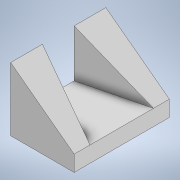
# Autodesk Inventor part: 零件9
Saved by Autodesk Inventor 2020 (Build 240168000, 168)
## iProperties
Created: 2020-09-19
Part Number: 零件9
Material: 一般
Document SubType Name: Modeling
Designer: User
Density: 1 g/cm^3
Appearance: 預設
Author: User
Autodesk Inventor part; units mm, degrees
ref_plane "YZ Plane" through (0, 0, 0) normal (1, 0, 0) x (0, 1, 0)
ref_plane "XZ Plane" through (0, 0, 0) normal (0, 1, 0) x (-1, 0, 0)
ref_plane "XY Plane" through (0, 0, 0) normal (0, 0, 1) x (1, 0, 0)
sketch "草圖1" plane through (0, 0, 0) normal (0, 1, 0) x (-1, 0, 0)
  line L0 (0, 0) -> (40, 0)
  line L1 (40, 0) -> (40, -60)
  line L2 (40, -60) -> (0, -60)
  line L3 (0, -60) -> (0, 0)
  line L4 (40, -20) -> (0, -10)
  line L5 (40, -40) -> (0, -50)
  dimension "d0" = 40
  dimension "d1" = 60
  dimension "d2" = 20
  dimension "d3" = 20
  dimension "d4" = 10
  dimension "d5" = 10
  constraints: 12 end point, 4 point on line, 2 parallel, 1 horizontal, 1 perpendicular
  measures "d0" distance of L1.end L2.end
  measures "d1" distance of L0.end L1.end
  measures "d2" distance of L4.start L0.end
  measures "d3" distance of L1.end L5.start
  measures "d4" distance of L4.end L0.start
  measures "d5" distance from line of L2 L5.end
extrude "擠出1" add sketch "草圖1" along normal blind 40 contours L0 L1 L4 L3 | L5 L1 L2 L3
extrude "擠出2" add sketch "草圖1" along normal blind 10 contours L4 L1 L5 L3
sketch "草圖2" plane through (0, 0, -60) normal (0, 0, -1) x (-1, 0, 0)
  line L0 (0, 0) -> (0, 40) projected
  line L1 (0, 40) -> (0, 10)
  line L2 (40, 0) -> (40, 40) projected
  line L3 (0, 10) -> (40, 40)
  line L4 (40, 40) -> (0, 40)
  dimension "d10" = 30
  constraints: 6 end point, 1 perpendicular, 1 point on line
  measures "d10" distance of L0.end L1.end
extrude "擠出3" cut sketch "草圖2" against normal blind 60
